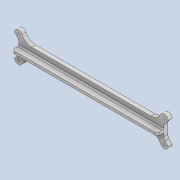
# Autodesk Inventor part: test_bridge_1
Saved by Autodesk Inventor 2020 (Build 240168000, 168)
## iProperties
Created: 2022-01-22
Part Number: test_bridge_1
Material: Generic
Document SubType Name: Modeling
Designer: Shuang Peng
Density: 1 g/cm^3
Appearance: Default
Author: Shuang Peng
Autodesk Inventor part; units mm, degrees
ref_plane "YZ Plane" through (0, 0, 0) normal (1, 0, 0) x (0, 1, 0)
ref_plane "XZ Plane" through (0, 0, 0) normal (0, 1, 0) x (-1, 0, 0)
ref_plane "XY Plane" through (0, 0, 0) normal (0, 0, 1) x (1, 0, 0)
sketch "Sketch1" plane through (0, 0, 0) normal (0, 0, 1) x (1, 0, 0)
  circle A0 centre (-126.3, 8.5) radius 0.95 projected
  circle A1 centre (-126.3, -8.5) radius 0.95 projected
  circle A2 centre (-15.7, -8.5) radius 0.95 projected
  circle A3 centre (-15.7, 8.5) radius 0.95 projected
  line L0 (-21, 18) -> (-21, -18) projected
  line L1 (-121, -18) -> (-121, 18) projected
  line L2 (-121, 0) -> (-21, 0)
  line L3 (-126, 5) -> (-126, -5)
  line L4 (-126, -5) -> (-16, -5)
  line L5 (-16, -5) -> (-16, 5)
  line L6 (-16, 5) -> (-126, 5)
  line L7 (-126, 5) -> (-16, -5) construction
  line L8 (-126, -5) -> (-16, 5) construction
  line L9 (-126.3, 8.5) -> (-126.3, -8.5) construction
  line L10 (-129.3, 8.5) -> (-129.3, -8.5)
  line L11 (-123.3, -8.5) -> (-123.3, 8.5)
  arc A4 (-123.3, 8.5) -> (-129.3, 8.5) centre (-126.3, 8.5) ccw
  arc A5 (-129.3, -8.5) -> (-123.3, -8.5) centre (-126.3, -8.5) ccw
  line L12 (-15.7, 8.5) -> (-15.7, -8.5) construction
  line L13 (-18.7, 8.5) -> (-18.7, -8.5)
  line L14 (-12.7, -8.5) -> (-12.7, 8.5)
  arc A6 (-12.7, 8.5) -> (-18.7, 8.5) centre (-15.7, 8.5) ccw
  arc A7 (-18.7, -8.5) -> (-12.7, -8.5) centre (-15.7, -8.5) ccw
  line L15 (-16, 5) -> (-12.7, 8.5)
  line L16 (-16, -5) -> (-12.7, -8.5)
  line L17 (-126, 5) -> (-129.3, 8.5)
  line L18 (-126, -5) -> (-129.3, -8.5)
  point P0 (0, 0)
  point P1 (-71, 0)
  point P2 (-126.3, 0)
  point P3 (-15.7, 0)
  point P4 (-123.3, 5)
  point P5 (-123.3, -5)
  point P6 (-18.7, -5)
  point P7 (-18.7, 5)
  dimension "d0" = 10
  dimension "d1" = 110
  dimension "d2" = 6
  dimension "d3" = 6
  constraints: 38 end point, 8 point on circle, 8 tangent, 7 midpoint, 4 centre point, 4 parallel, 2 perpendicular, 2 vertical
  measures "d0" distance of L3.start L3.end
  measures "d1" distance of L4.end L3.end
  measures "d2" diameter of A5
  measures "d3" diameter of A7
extrude "Extrusion1" add sketch "Sketch1" along normal blind 3 contours L6 L13 L4 L0 | L0 L2 L1 L6 | L0 L4 L1 L2 | L13 A6 L15 L6 | L6 L5 L4 L13 | L1 L4 L11 L6 | L4 L16 A7 L13 | L11 L4 L3 L6 | L6 L17 A4 L11 | L11 A5 L18 L4
fillet "Fillet1" radius 8 4 edges at (-123.3, 5, 1.5) (-123.3, -5, 1.5) (-18.7, -5, 1.5) (-18.7, 5, 1.5)
fillet "Fillet2" radius 3 4 edges at (-126, 5, 1.5) (-126, -5, 1.5) (-16, 5, 1.5) (-16, -5, 1.5)
sketch "Sketch2" plane through (0, 0, 3) normal (0, 0, 1) x (1, 0, 0)
  arc A0 (-18.4375, -9.7273) -> (-12.7, -8.5) centre (-15.7, -8.5) ccw projected
  line L0 (-12.7, -8.5) -> (-15.1828, -5.8668) projected
  arc A1 (-16, -3.8087) -> (-15.1828, -5.8668) centre (-13, -3.8087) ccw projected
  line L1 (-16, -3.8087) -> (-16, 3.8087) projected
  arc A2 (-15.1828, 5.8668) -> (-16, 3.8087) centre (-13, 3.8087) ccw projected
  line L2 (-15.1828, 5.8668) -> (-12.7, 8.5) projected
  arc A3 (-12.7, 8.5) -> (-18.4375, 9.7273) centre (-15.7, 8.5) ccw projected
  arc A4 (-25.7374, 5) -> (-18.4375, 9.7273) centre (-25.7374, 13) ccw projected
  line L3 (-25.7374, 5) -> (-116.2626, 5) projected
  arc A5 (-123.5625, 9.7273) -> (-116.2626, 5) centre (-116.2626, 13) ccw projected
  arc A6 (-123.5625, 9.7273) -> (-129.3, 8.5) centre (-126.3, 8.5) ccw projected
  line L4 (-129.3, 8.5) -> (-126.8172, 5.8668) projected
  arc A7 (-126, 3.8087) -> (-126.8172, 5.8668) centre (-129, 3.8087) ccw projected
  line L5 (-126, 3.8087) -> (-126, -3.8087) projected
  arc A8 (-126.8172, -5.8668) -> (-126, -3.8087) centre (-129, -3.8087) ccw projected
  line L6 (-126.8172, -5.8668) -> (-129.3, -8.5) projected
  arc A9 (-129.3, -8.5) -> (-123.5625, -9.7273) centre (-126.3, -8.5) ccw projected
  arc A10 (-116.2626, -5) -> (-123.5625, -9.7273) centre (-116.2626, -13) ccw projected
  line L7 (-116.2626, -5) -> (-25.7374, -5) projected
  arc A11 (-18.4375, -9.7273) -> (-25.7374, -5) centre (-25.7374, -13) ccw projected
  circle A12 centre (-15.7, 8.5) radius 0.95 projected
  circle A13 centre (-15.7, -8.5) radius 0.95 projected
  circle A14 centre (-126.3, -8.5) radius 0.95 projected
  circle A15 centre (-126.3, 8.5) radius 0.95 projected
  line L8 (-126, 3.8087) -> (-126, -3.8087) projected
  line L9 (-126, 0) -> (-16, 0)
  line L10 (-126, 1) -> (-126, -1)
  line L11 (-126, -1) -> (-16, -1)
  line L12 (-16, -1) -> (-16, 1)
  line L13 (-16, 1) -> (-126, 1)
  line L14 (-126, 1) -> (-16, -1) construction
  line L15 (-126, -1) -> (-16, 1) construction
  line L16 (-16, -3.8087) -> (-16, 3.8087) projected
  point P0 (0, 0)
  point P1 (-71, 0)
  dimension "d8" = 2
  constraints: 14 end point, 5 midpoint, 2 parallel, 2 perpendicular, 1 point on line
  measures "d8" distance of L10.start L10.end
extrude "Extrusion2" add sketch "Sketch2" along normal blind 5 contours L11 L5 L9 L1 | L9 L5 L13 L1
fillet "Fillet3" radius 1 2 edges at (-71, -1, 3) (-71, 1, 3)
fillet "Fillet4" radius 2 2 edges at (-126, 0, 8) (-16, 0, 8)
body "Solid1"
